Autodesk Fusion 360 part; units mm, degrees
(part 8 of 8)
  spline S32 degree 5 poles (83.4638, 120.4328) (83.5006, 120.4863) (83.5729, 120.594) (83.6772, 120.7581) (83.8082, 120.9817) (83.961, 121.2679) (84.106, 121.5588) (84.2462, 121.8526) (84.3838, 122.1479) (84.5197, 122.4443) (84.6536, 122.7417) (84.7851, 123.0405) (84.9132, 123.3412) (85.0374, 123.644) (85.1577, 123.949) (85.2744, 124.2559) (85.3881, 124.5645) (85.4991, 124.8744) (85.608, 125.1854) (85.7147, 125.4975) (85.8192, 125.8106) (85.9214, 126.1249) (86.0213, 126.4403) (86.1187, 126.757) (86.2136, 127.0748) (86.3062, 127.3938) (86.3966, 127.7138) (86.4849, 128.0348) (86.5711, 128.3567) (86.6553, 128.6794) (86.7376, 129.0031) (86.8178, 129.3277) (86.896, 129.6531) (86.9723, 129.9794) (87.0465, 130.3066) (87.1189, 130.6346) (87.1893, 130.9633) (87.2578, 131.2929) (87.3245, 131.6232) (87.3894, 131.9542) (87.4525, 132.286) (87.5137, 132.6184) (87.5732, 132.9516) (87.6309, 133.2854) (87.6869, 133.6199) (87.7411, 133.9551) (87.7935, 134.2909) (87.8443, 134.6274) (87.8933, 134.9645) (87.9407, 135.3021) (87.9864, 135.6404) (88.0305, 135.9792) (88.0729, 136.3187) (88.1136, 136.6587) (88.1527, 136.9992) (88.1902, 137.3403) (88.2261, 137.6819) (88.2604, 138.024) (88.2931, 138.3667) (88.3243, 138.7098) (88.3538, 139.0535) (88.3818, 139.3976) (88.4082, 139.7422) (88.4331, 140.0873) (88.4565, 140.4328) (88.4783, 140.7788) (88.4986, 141.1253) (88.5174, 141.4721) (88.5347, 141.8194) (88.5504, 142.1671) (88.5647, 142.5153) (88.575, 142.7941) (88.582, 143.0034) (88.5864, 143.143) (88.5885, 143.2129) knots 0 0 0 0 0 0 0.01428571 0.02857143 0.04285714 0.05714286 0.07142857 0.08571429 0.1 0.11428571 0.12857143 0.14285714 0.15714286 0.17142857 0.18571429 0.2 0.21428571 0.22857143 0.24285714 0.25714286 0.27142857 0.28571429 0.3 0.31428571 0.32857143 0.34285714 0.35714286 0.37142857 0.38571429 0.4 0.41428571 0.42857143 0.44285714 0.45714286 0.47142857 0.48571429 0.5 0.51428571 0.52857143 0.54285714 0.55714286 0.57142857 0.58571429 0.6 0.61428571 0.62857143 0.64285714 0.65714286 0.67142857 0.68571429 0.7 0.71428571 0.72857143 0.74285714 0.75714286 0.77142857 0.78571429 0.8 0.81428571 0.82857143 0.84285714 0.85714286 0.87142857 0.88571429 0.9 0.91428571 0.92857143 0.94285714 0.95714286 0.97142857 0.98571429 1 1 1 1 1 1
  arc A66 (88.5885, 143.2129) -> (80.7195, 147.756) centre (2.1352, 2.5578) ccw
  spline S33 degree 5 poles (80.7195, 147.756) (80.66, 147.7193) (80.5413, 147.6457) (80.3635, 147.535) (80.1272, 147.3867) (79.8328, 147.2003) (79.5396, 147.0127) (79.2475, 146.8241) (78.9565, 146.6344) (78.6666, 146.4436) (78.3779, 146.2517) (78.0903, 146.0587) (77.8039, 145.8646) (77.5187, 145.6694) (77.2347, 145.4731) (76.9518, 145.2757) (76.6702, 145.0772) (76.3898, 144.8775) (76.1107, 144.6768) (75.8328, 144.4749) (75.5561, 144.2718) (75.2808, 144.0677) (75.0067, 143.8624) (74.734, 143.656) (74.4625, 143.4484) (74.1924, 143.2397) (73.9237, 143.0298) (73.6563, 142.8188) (73.3903, 142.6066) (73.1257, 142.3933) (72.8626, 142.1788) (72.6008, 141.963) (72.3406, 141.7462) (72.0818, 141.5281) (71.8245, 141.3088) (71.5687, 141.0883) (71.3145, 140.8666) (71.0618, 140.6437) (70.8107, 140.4195) (70.5611, 140.1942) (70.3133, 139.9676) (70.0671, 139.7397) (69.8226, 139.5105) (69.5799, 139.28) (69.3389, 139.0483) (69.0997, 138.8152) (68.8623, 138.5809) (68.6266, 138.3452) (68.3928, 138.1083) (68.1608, 137.87) (67.9309, 137.6303) (67.7032, 137.3892) (67.4776, 137.1465) (67.2544, 136.9023) (67.0333, 136.6567) (66.8144, 136.4096) (66.5975, 136.1611) (66.3825, 135.9114) (66.1697, 135.6602) (65.9593, 135.4075) (65.7519, 135.153) (65.5479, 134.8963) (65.3477, 134.6373) (65.1514, 134.376) (64.9583, 134.1128) (64.7677, 133.8481) (64.579, 133.5822) (64.392, 133.3154) (64.2077, 133.0471) (64.0283, 132.776) (63.8569, 132.5006) (63.7287, 132.2754) (63.6387, 132.103) (63.5816, 131.9866) (63.5537, 131.9279) knots -1 -1 -1 -1 -1 -1 -0.98571429 -0.97142857 -0.95714286 -0.94285714 -0.92857143 -0.91428571 -0.9 -0.88571429 -0.87142857 -0.85714286 -0.84285714 -0.82857143 -0.81428571 -0.8 -0.78571429 -0.77142857 -0.75714286 -0.74285714 -0.72857143 -0.71428571 -0.7 -0.68571429 -0.67142857 -0.65714286 -0.64285714 -0.62857143 -0.61428571 -0.6 -0.58571429 -0.57142857 -0.55714286 -0.54285714 -0.52857143 -0.51428571 -0.5 -0.48571429 -0.47142857 -0.45714286 -0.44285714 -0.42857143 -0.41428571 -0.4 -0.38571429 -0.37142857 -0.35714286 -0.34285714 -0.32857143 -0.31428571 -0.3 -0.28571429 -0.27142857 -0.25714286 -0.24285714 -0.22857143 -0.21428571 -0.2 -0.18571429 -0.17142857 -0.15714286 -0.14285714 -0.12857143 -0.11428571 -0.1 -0.08571429 -0.07142857 -0.05714286 -0.04285714 -0.02857143 -0.01428571 0 0 0 0 0 0
  line L33 (63.5537, 131.9279) -> (61.6139, 127.8434)
  arc A67 (59.5156, 127.0826) -> (61.6139, 127.8434) centre (60.1799, 128.5244) ccw
  arc A68 (59.5156, 127.0826) -> (49.6135, 131.1842) centre (2.1352, 2.5578) ccw
  arc A69 (48.6677, 133.2059) -> (49.6135, 131.1842) centre (50.1633, 132.6735) ccw
  line L34 (48.6677, 133.2059) -> (50.1843, 137.4657)
  spline S34 degree 5 poles (50.1843, 137.4657) (50.2061, 137.5269) (50.248, 137.6496) (50.3062, 137.8351) (50.3749, 138.085) (50.4484, 138.401) (50.5132, 138.7195) (50.5726, 139.0396) (50.6291, 139.3605) (50.6836, 139.6819) (50.736, 140.0039) (50.7856, 140.3265) (50.8315, 140.6501) (50.8731, 140.9748) (50.9104, 141.3005) (50.9437, 141.6272) (50.9736, 141.9546) (51.0007, 142.2827) (51.0253, 142.6113) (51.0476, 142.9404) (51.0675, 143.2699) (51.085, 143.5999) (51.0998, 143.9305) (51.1119, 144.2615) (51.1213, 144.5931) (51.1282, 144.9252) (51.1327, 145.2576) (51.1349, 145.5905) (51.1349, 145.9238) (51.1327, 146.2574) (51.1284, 146.5913) (51.1219, 146.9256) (51.1132, 147.2602) (51.1024, 147.5951) (51.0894, 147.9303) (51.0744, 148.2658) (51.0573, 148.6016) (51.0383, 148.9377) (51.0172, 149.274) (50.9942, 149.6105) (50.9692, 149.9473) (50.9424, 150.2843) (50.9136, 150.6215) (50.8829, 150.9589) (50.8504, 151.2965) (50.816, 151.6343) (50.7797, 151.9722) (50.7417, 152.3104) (50.7018, 152.6486) (50.6602, 152.9871) (50.6168, 153.3256) (50.5716, 153.6643) (50.5247, 154.0032) (50.4761, 154.3421) (50.4258, 154.6812) (50.3737, 155.0203) (50.32, 155.3596) (50.2645, 155.699) (50.2074, 156.0384) (50.1487, 156.3779) (50.0883, 156.7175) (50.0263, 157.0572) (49.9626, 157.3969) (49.8973, 157.7366) (49.8305, 158.0765) (49.762, 158.4163) (49.6919, 158.7562) (49.6203, 159.0961) (49.5471, 159.436) (49.4724, 159.776) (49.3961, 160.1159) (49.3338, 160.3879) (49.2864, 160.5919) (49.2545, 160.7279) (49.2384, 160.7959) knots 0 0 0 0 0 0 0.01428571 0.02857143 0.04285714 0.05714286 0.07142857 0.08571429 0.1 0.11428571 0.12857143 0.14285714 0.15714286 0.17142857 0.18571429 0.2 0.21428571 0.22857143 0.24285714 0.25714286 0.27142857 0.28571429 0.3 0.31428571 0.32857143 0.34285714 0.35714286 0.37142857 0.38571429 0.4 0.41428571 0.42857143 0.44285714 0.45714286 0.47142857 0.48571429 0.5 0.51428571 0.52857143 0.54285714 0.55714286 0.57142857 0.58571429 0.6 0.61428571 0.62857143 0.64285714 0.65714286 0.67142857 0.68571429 0.7 0.71428571 0.72857143 0.74285714 0.75714286 0.77142857 0.78571429 0.8 0.81428571 0.82857143 0.84285714 0.85714286 0.87142857 0.88571429 0.9 0.91428571 0.92857143 0.94285714 0.95714286 0.97142857 0.98571429 1 1 1 1 1 1
  arc A70 (49.2384, 160.7959) -> (40.4617, 163.1476) centre (2.1352, 2.5578) ccw
  spline S35 degree 5 poles (40.4617, 163.1476) (40.4138, 163.0968) (40.3182, 162.9949) (40.1751, 162.842) (39.9852, 162.6376) (39.7491, 162.3813) (39.5144, 162.1243) (39.2811, 161.8665) (39.0491, 161.6079) (38.8185, 161.3486) (38.5893, 161.0885) (38.3614, 160.8277) (38.135, 160.5661) (37.91, 160.3037) (37.6865, 160.0406) (37.4644, 159.7767) (37.2438, 159.512) (37.0246, 159.2466) (36.8069, 158.9804) (36.5907, 158.7135) (36.3761, 158.4458) (36.1629, 158.1773) (35.9514, 157.9081) (35.7413, 157.6381) (35.5329, 157.3674) (35.326, 157.0959) (35.1207, 156.8236) (34.9171, 156.5506) (34.7151, 156.2768) (34.5147, 156.0022) (34.316, 155.7269) (34.119, 155.4508) (33.9238, 155.1739) (33.7302, 154.8963) (33.5385, 154.6179) (33.3485, 154.3387) (33.1603, 154.0587) (32.9739, 153.778) (32.7893, 153.4965) (32.6067, 153.2143) (32.4259, 152.9312) (32.2471, 152.6474) (32.0702, 152.3627) (31.8954, 152.0773) (31.7227, 151.791) (31.5519, 151.504) (31.3832, 151.2162) (31.2166, 150.9276) (31.0521, 150.6382) (30.8897, 150.3481) (30.7297, 150.057) (30.5721, 149.7652) (30.417, 149.4724) (30.2646, 149.1787) (30.1146, 148.8842) (29.9671, 148.5889) (29.8219, 148.2928) (29.6789, 147.9959) (29.5383, 147.6982) (29.4005, 147.3997) (29.266, 147.1001) (29.1355, 146.7994) (29.0091, 146.4974) (28.8871, 146.1942) (28.7687, 145.89) (28.6532, 145.5849) (28.5397, 145.2793) (28.4281, 144.9732) (28.3195, 144.6663) (28.2164, 144.3581) (28.1221, 144.0477) (28.0566, 143.7969) (28.0142, 143.6072) (27.9892, 143.4799) (27.9775, 143.416) knots -1 -1 -1 -1 -1 -1 -0.98571429 -0.97142857 -0.95714286 -0.94285714 -0.92857143 -0.91428571 -0.9 -0.88571429 -0.87142857 -0.85714286 -0.84285714 -0.82857143 -0.81428571 -0.8 -0.78571429 -0.77142857 -0.75714286 -0.74285714 -0.72857143 -0.71428571 -0.7 -0.68571429 -0.67142857 -0.65714286 -0.64285714 -0.62857143 -0.61428571 -0.6 -0.58571429 -0.57142857 -0.55714286 -0.54285714 -0.52857143 -0.51428571 -0.5 -0.48571429 -0.47142857 -0.45714286 -0.44285714 -0.42857143 -0.41428571 -0.4 -0.38571429 -0.37142857 -0.35714286 -0.34285714 -0.32857143 -0.31428571 -0.3 -0.28571429 -0.27142857 -0.25714286 -0.24285714 -0.22857143 -0.21428571 -0.2 -0.18571429 -0.17142857 -0.15714286 -0.14285714 -0.12857143 -0.11428571 -0.1 -0.08571429 -0.07142857 -0.05714286 -0.04285714 -0.02857143 -0.01428571 0 0 0 0 0 0
  line L35 (27.9775, 143.416) -> (27.1609, 138.9686)
  arc A71 (25.331, 137.6907) -> (27.1609, 138.9686) centre (25.5995, 139.2553) ccw
  arc A72 (25.331, 137.6907) -> (14.7048, 139.0896) centre (2.1352, 2.5578) ccw
  arc A73 (13.2679, 140.7977) -> (14.7048, 139.0896) centre (14.8503, 140.6704) ccw
  line L36 (13.2679, 140.7977) -> (13.6303, 145.3049)
  spline S36 degree 5 poles (13.6303, 145.3049) (13.6355, 145.3696) (13.6443, 145.499) (13.6525, 145.6932) (13.6541, 145.9524) (13.6434, 146.2766) (13.6235, 146.6011) (13.598, 146.9256) (13.5696, 147.2502) (13.539, 147.5748) (13.5063, 147.8993) (13.4707, 148.2238) (13.4313, 148.5483) (13.3875, 148.8726) (13.3392, 149.1969) (13.2868, 149.5211) (13.231, 149.8451) (13.1722, 150.169) (13.1109, 150.4928) (13.0473, 150.8164) (12.9813, 151.1399) (12.9127, 151.4631) (12.8414, 151.7863) (12.7674, 152.1092) (12.6907, 152.4319) (12.6115, 152.7544) (12.5297, 153.0768) (12.4457, 153.3989) (12.3594, 153.7207) (12.271, 154.0424) (12.1804, 154.3638) (12.0876, 154.685) (11.9926, 155.006) (11.8955, 155.3267) (11.7962, 155.6472) (11.6948, 155.9673) (11.5914, 156.2873) (11.486, 156.6069) (11.3786, 156.9263) (11.2693, 157.2455) (11.158, 157.5643) (11.0449, 157.8829) (10.9298, 158.2011) (10.8129, 158.5191) (10.694, 158.8368) (10.5734, 159.1541) (10.4509, 159.4712) (10.3267, 159.7879) (10.2006, 160.1044) (10.0728, 160.4205) (9.9433, 160.7363) (9.812, 161.0518) (9.679, 161.3669) (9.5443, 161.6817) (9.4079, 161.9962) (9.2698, 162.3104) (9.1301, 162.6241) (8.9887, 162.9376) (8.8457, 163.2507) (8.7011, 163.5634) (8.5549, 163.8758) (8.407, 164.1878) (8.2576, 164.4995) (8.1066, 164.8108) (7.9541, 165.1217) (7.8, 165.4323) (7.6444, 165.7424) (7.4872, 166.0522) (7.3285, 166.3616) (7.1683, 166.6706) (7.0066, 166.9793) (6.8761, 167.2259) (6.7775, 167.4106) (6.7115, 167.5338) (6.6784, 167.5953) knots 0 0 0 0 0 0 0.01428571 0.02857143 0.04285714 0.05714286 0.07142857 0.08571429 0.1 0.11428571 0.12857143 0.14285714 0.15714286 0.17142857 0.18571429 0.2 0.21428571 0.22857143 0.24285714 0.25714286 0.27142857 0.28571429 0.3 0.31428571 0.32857143 0.34285714 0.35714286 0.37142857 0.38571429 0.4 0.41428571 0.42857143 0.44285714 0.45714286 0.47142857 0.48571429 0.5 0.51428571 0.52857143 0.54285714 0.55714286 0.57142857 0.58571429 0.6 0.61428571 0.62857143 0.64285714 0.65714286 0.67142857 0.68571429 0.7 0.71428571 0.72857143 0.74285714 0.75714286 0.77142857 0.78571429 0.8 0.81428571 0.82857143 0.84285714 0.85714286 0.87142857 0.88571429 0.9 0.91428571 0.92857143 0.94285714 0.95714286 0.97142857 0.98571429 1 1 1 1 1 1
  arc A74 (6.6784, 167.5953) -> (-2.4079, 167.5953) centre (2.1352, 2.5578) ccw
  spline S37 degree 5 poles (-2.4079, 167.5953) (-2.441, 167.5338) (-2.5071, 167.4106) (-2.6056, 167.2259) (-2.7362, 166.9793) (-2.8979, 166.6706) (-3.0581, 166.3616) (-3.2167, 166.0522) (-3.3739, 165.7424) (-3.5295, 165.4323) (-3.6836, 165.1217) (-3.8362, 164.8108) (-3.9872, 164.4995) (-4.1366, 164.1878) (-4.2844, 163.8758) (-4.4306, 163.5634) (-4.5753, 163.2507) (-4.7183, 162.9376) (-4.8596, 162.6241) (-4.9994, 162.3104) (-5.1374, 161.9962) (-5.2738, 161.6817) (-5.4085, 161.3669) (-5.5415, 161.0518) (-5.6728, 160.7363) (-5.8024, 160.4205) (-5.9302, 160.1044) (-6.0562, 159.7879) (-6.1805, 159.4712) (-6.3029, 159.1541) (-6.4236, 158.8368) (-6.5424, 158.5191) (-6.6594, 158.2011) (-6.7744, 157.8829) (-6.8876, 157.5643) (-6.9989, 157.2455) (-7.1082, 156.9263) (-7.2156, 156.6069) (-7.321, 156.2873) (-7.4244, 155.9673) (-7.5257, 155.6472) (-7.625, 155.3267) (-7.7221, 155.006) (-7.8171, 154.685) (-7.9099, 154.3638) (-8.0005, 154.0424) (-8.089, 153.7207) (-8.1753, 153.3989) (-8.2593, 153.0768) (-8.341, 152.7544) (-8.4203, 152.4319) (-8.497, 152.1092) (-8.571, 151.7863) (-8.6422, 151.4631) (-8.7108, 151.1399) (-8.7768, 150.8164) (-8.8405, 150.4928) (-8.9017, 150.169) (-8.9605, 149.8451) (-9.0164, 149.5211) (-9.0687, 149.1969) (-9.117, 148.8726) (-9.1609, 148.5483) (-9.2003, 148.2238) (-9.2359, 147.8993) (-9.2686, 147.5748) (-9.2991, 147.2502) (-9.3276, 146.9256) (-9.3531, 146.6011) (-9.3729, 146.2766) (-9.3837, 145.9524) (-9.382, 145.6932) (-9.3738, 145.499) (-9.3651, 145.3696) (-9.3599, 145.3049) knots -1 -1 -1 -1 -1 -1 -0.98571429 -0.97142857 -0.95714286 -0.94285714 -0.92857143 -0.91428571 -0.9 -0.88571429 -0.87142857 -0.85714286 -0.84285714 -0.82857143 -0.81428571 -0.8 -0.78571429 -0.77142857 -0.75714286 -0.74285714 -0.72857143 -0.71428571 -0.7 -0.68571429 -0.67142857 -0.65714286 -0.64285714 -0.62857143 -0.61428571 -0.6 -0.58571429 -0.57142857 -0.55714286 -0.54285714 -0.52857143 -0.51428571 -0.5 -0.48571429 -0.47142857 -0.45714286 -0.44285714 -0.42857143 -0.41428571 -0.4 -0.38571429 -0.37142857 -0.35714286 -0.34285714 -0.32857143 -0.31428571 -0.3 -0.28571429 -0.27142857 -0.25714286 -0.24285714 -0.22857143 -0.21428571 -0.2 -0.18571429 -0.17142857 -0.15714286 -0.14285714 -0.12857143 -0.11428571 -0.1 -0.08571429 -0.07142857 -0.05714286 -0.04285714 -0.02857143 -0.01428571 0 0 0 0 0 0
  line L37 (-9.3599, 145.3049) -> (-8.9975, 140.7977)
  arc A75 (-10.4344, 139.0896) -> (-8.9975, 140.7977) centre (-10.5799, 140.6704) ccw
  arc A76 (-10.4344, 139.0896) -> (-21.0605, 137.6907) centre (2.1352, 2.5578) ccw
  arc A77 (-22.8905, 138.9686) -> (-21.0605, 137.6907) centre (-21.3291, 139.2553) ccw
  line L38 (-22.8905, 138.9686) -> (-23.707, 143.416)
  spline S38 degree 5 poles (-23.707, 143.416) (-23.7188, 143.4799) (-23.7438, 143.6072) (-23.7861, 143.7969) (-23.8516, 144.0477) (-23.9459, 144.3581) (-24.0491, 144.6663) (-24.1577, 144.9732) (-24.2692, 145.2793) (-24.3827, 145.5849) (-24.4983, 145.89) (-24.6166, 146.1942) (-24.7387, 146.4974) (-24.865, 146.7994) (-24.9956, 147.1001) (-25.1301, 147.3997) (-25.2679, 147.6982) (-25.4085, 147.9959) (-25.5515, 148.2928) (-25.6967, 148.5889) (-25.8442, 148.8842) (-25.9941, 149.1787) (-26.1466, 149.4724) (-26.3016, 149.7652) (-26.4592, 150.057) (-26.6192, 150.3481) (-26.7816, 150.6382) (-26.9462, 150.9276) (-27.1128, 151.2162) (-27.2815, 151.504) (-27.4522, 151.791) (-27.625, 152.0773) (-27.7998, 152.3627) (-27.9766, 152.6474) (-28.1554, 152.9312) (-28.3362, 153.2143) (-28.5189, 153.4965) (-28.7035, 153.778) (-28.8898, 154.0587) (-29.078, 154.3387) (-29.268, 154.6179) (-29.4598, 154.8963) (-29.6533, 155.1739) (-29.8486, 155.4508) (-30.0456, 155.7269) (-30.2442, 156.0022) (-30.4446, 156.2768) (-30.6466, 156.5506) (-30.8503, 156.8236) (-31.0555, 157.0959) (-31.2624, 157.3674) (-31.4709, 157.6381) (-31.6809, 157.9081) (-31.8925, 158.1773) (-32.1056, 158.4458) (-32.3203, 158.7135) (-32.5365, 158.9804) (-32.7541, 159.2466) (-32.9733, 159.512) (-33.1939, 159.7767) (-33.416, 160.0406) (-33.6396, 160.3037) (-33.8646, 160.5661) (-34.091, 160.8277) (-34.3188, 161.0885) (-34.548, 161.3486) (-34.7786, 161.6079) (-35.0106, 161.8665) (-35.244, 162.1243) (-35.4787, 162.3813) (-35.7148, 162.6376) (-35.9047, 162.842) (-36.0477, 162.9949) (-36.1434, 163.0968) (-36.1913, 163.1476) knots 0 0 0 0 0 0 0.01428571 0.02857143 0.04285714 0.05714286 0.07142857 0.08571429 0.1 0.11428571 0.12857143 0.14285714 0.15714286 0.17142857 0.18571429 0.2 0.21428571 0.22857143 0.24285714 0.25714286 0.27142857 0.28571429 0.3 0.31428571 0.32857143 0.34285714 0.35714286 0.37142857 0.38571429 0.4 0.41428571 0.42857143 0.44285714 0.45714286 0.47142857 0.48571429 0.5 0.51428571 0.52857143 0.54285714 0.55714286 0.57142857 0.58571429 0.6 0.61428571 0.62857143 0.64285714 0.65714286 0.67142857 0.68571429 0.7 0.71428571 0.72857143 0.74285714 0.75714286 0.77142857 0.78571429 0.8 0.81428571 0.82857143 0.84285714 0.85714286 0.87142857 0.88571429 0.9 0.91428571 0.92857143 0.94285714 0.95714286 0.97142857 0.98571429 1 1 1 1 1 1
  arc A78 (-36.1913, 163.1476) -> (-44.968, 160.7959) centre (2.1352, 2.5578) ccw
  spline S39 degree 5 poles (-44.968, 160.7959) (-44.984, 160.7279) (-45.0159, 160.5919) (-45.0633, 160.3879) (-45.1256, 160.1159) (-45.2019, 159.776) (-45.2767, 159.436) (-45.3499, 159.0961) (-45.4215, 158.7562) (-45.4915, 158.4163) (-45.56, 158.0765) (-45.6269, 157.7366) (-45.6922, 157.3969) (-45.7558, 157.0572) (-45.8178, 156.7175) (-45.8782, 156.3779) (-45.937, 156.0384) (-45.9941, 155.699) (-46.0495, 155.3596) (-46.1033, 155.0203) (-46.1553, 154.6812) (-46.2057, 154.3421) (-46.2543, 154.0032) (-46.3012, 153.6643) (-46.3464, 153.3256) (-46.3898, 152.9871) (-46.4314, 152.6486) (-46.4712, 152.3104) (-46.5093, 151.9722) (-46.5455, 151.6343) (-46.5799, 151.2965) (-46.6125, 150.9589) (-46.6431, 150.6215) (-46.6719, 150.2843) (-46.6988, 149.9473) (-46.7237, 149.6105) (-46.7467, 149.274) (-46.7678, 148.9377) (-46.7869, 148.6016) (-46.804, 148.2658) (-46.819, 147.9303) (-46.8319, 147.5951) (-46.8427, 147.2602) (-46.8514, 146.9256) (-46.8579, 146.5913) (-46.8623, 146.2574) (-46.8644, 145.9238) (-46.8645, 145.5905) (-46.8623, 145.2576) (-46.8578, 144.9252) (-46.8509, 144.5931) (-46.8414, 144.2615) (-46.8293, 143.9305) (-46.8145, 143.5999) (-46.7971, 143.2699) (-46.7772, 142.9404) (-46.7549, 142.6113) (-46.7303, 142.2827) (-46.7032, 141.9546) (-46.6733, 141.6272) (-46.6399, 141.3005) (-46.6027, 140.9748) (-46.5611, 140.6501) (-46.5152, 140.3265) (-46.4656, 140.0039) (-46.4131, 139.6819) (-46.3586, 139.3605) (-46.3021, 139.0396) (-46.2427, 138.7195) (-46.178, 138.401) (-46.1044, 138.085) (-46.0358, 137.8351) (-45.9776, 137.6496) (-45.9356, 137.5269) (-45.9138, 137.4657) knots -1 -1 -1 -1 -1 -1 -0.98571429 -0.97142857 -0.95714286 -0.94285714 -0.92857143 -0.91428571 -0.9 -0.88571429 -0.87142857 -0.85714286 -0.84285714 -0.82857143 -0.81428571 -0.8 -0.78571429 -0.77142857 -0.75714286 -0.74285714 -0.72857143 -0.71428571 -0.7 -0.68571429 -0.67142857 -0.65714286 -0.64285714 -0.62857143 -0.61428571 -0.6 -0.58571429 -0.57142857 -0.55714286 -0.54285714 -0.52857143 -0.51428571 -0.5 -0.48571429 -0.47142857 -0.45714286 -0.44285714 -0.42857143 -0.41428571 -0.4 -0.38571429 -0.37142857 -0.35714286 -0.34285714 -0.32857143 -0.31428571 -0.3 -0.28571429 -0.27142857 -0.25714286 -0.24285714 -0.22857143 -0.21428571 -0.2 -0.18571429 -0.17142857 -0.15714286 -0.14285714 -0.12857143 -0.11428571 -0.1 -0.08571429 -0.07142857 -0.05714286 -0.04285714 -0.02857143 -0.01428571 0 0 0 0 0 0
  line L39 (-45.9138, 137.4657) -> (-44.3973, 133.2059)
  arc A79 (-45.3431, 131.1842) -> (-44.3973, 133.2059) centre (-45.8928, 132.6735) ccw
  arc A80 (-45.3431, 131.1842) -> (-55.2451, 127.0826) centre (2.1352, 2.5578) ccw
  arc A81 (-57.3435, 127.8434) -> (-55.2451, 127.0826) centre (-55.9095, 128.5244) ccw
  line L40 (-57.3435, 127.8434) -> (-59.2833, 131.9279)
  spline S40 degree 5 poles (-59.2833, 131.9279) (-59.3111, 131.9866) (-59.3682, 132.103) (-59.4582, 132.2754) (-59.5864, 132.5006) (-59.7578, 132.776) (-59.9373, 133.0471) (-60.1216, 133.3154) (-60.3085, 133.5822) (-60.4973, 133.8481) (-60.6879, 134.1128) (-60.8809, 134.376) (-61.0773, 134.6373) (-61.2775, 134.8963) (-61.4814, 135.153) (-61.6889, 135.4075) (-61.8992, 135.6602) (-62.1121, 135.9114) (-62.327, 136.1611) (-62.544, 136.4096) (-62.7629, 136.6567) (-62.9839, 136.9023) (-63.2072, 137.1465) (-63.4327, 137.3892) (-63.6605, 137.6303) (-63.8904, 137.87) (-64.1223, 138.1083) (-64.3562, 138.3452) (-64.5918, 138.5809) (-64.8293, 138.8152) (-65.0685, 139.0483) (-65.3094, 139.28) (-65.5521, 139.5105) (-65.7966, 139.7397) (-66.0428, 139.9676) (-66.2907, 140.1942) (-66.5402, 140.4195) (-66.7913, 140.6437) (-67.044, 140.8666) (-67.2983, 141.0883) (-67.554, 141.3088) (-67.8113, 141.5281) (-68.0701, 141.7462) (-68.3304, 141.963) (-68.5921, 142.1788) (-68.8553, 142.3933) (-69.1199, 142.6066) (-69.3859, 142.8188) (-69.6532, 143.0298) (-69.922, 143.2397) (-70.1921, 143.4484) (-70.4635, 143.656) (-70.7363, 143.8624) (-71.0103, 144.0677) (-71.2857, 144.2718) (-71.5623, 144.4749) (-71.8402, 144.6768) (-72.1194, 144.8775) (-72.3998, 145.0772) (-72.6814, 145.2757) (-72.9642, 145.4731) (-73.2482, 145.6694) (-73.5335, 145.8646) (-73.8199, 146.0587) (-74.1074, 146.2517) (-74.3962, 146.4436) (-74.686, 146.6344) (-74.977, 146.8241) (-75.2692, 147.0127) (-75.5624, 147.2003) (-75.8567, 147.3867) (-76.0931, 147.535) (-76.2709, 147.6457) (-76.3896, 147.7193) (-76.449, 147.756) knots 0 0 0 0 0 0 0.01428571 0.02857143 0.04285714 0.05714286 0.07142857 0.08571429 0.1 0.11428571 0.12857143 0.14285714 0.15714286 0.17142857 0.18571429 0.2 0.21428571 0.22857143 0.24285714 0.25714286 0.27142857 0.28571429 0.3 0.31428571 0.32857143 0.34285714 0.35714286 0.37142857 0.38571429 0.4 0.41428571 0.42857143 0.44285714 0.45714286 0.47142857 0.48571429 0.5 0.51428571 0.52857143 0.54285714 0.55714286 0.57142857 0.58571429 0.6 0.61428571 0.62857143 0.64285714 0.65714286 0.67142857 0.68571429 0.7 0.71428571 0.72857143 0.74285714 0.75714286 0.77142857 0.78571429 0.8 0.81428571 0.82857143 0.84285714 0.85714286 0.87142857 0.88571429 0.9 0.91428571 0.92857143 0.94285714 0.95714286 0.97142857 0.98571429 1 1 1 1 1 1
  arc A82 (-76.449, 147.756) -> (-84.318, 143.2129) centre (2.1352, 2.5578) ccw
  spline S41 degree 5 poles (-84.318, 143.2129) (-84.3159, 143.143) (-84.3115, 143.0034) (-84.3045, 142.7941) (-84.2943, 142.5153) (-84.28, 142.1671) (-84.2642, 141.8194) (-84.2469, 141.4721) (-84.2281, 141.1253) (-84.2078, 140.7788) (-84.186, 140.4328) (-84.1627, 140.0873) (-84.1378, 139.7422) (-84.1113, 139.3976) (-84.0834, 139.0535) (-84.0538, 138.7098) (-84.0227, 138.3667) (-83.99, 138.024) (-83.9557, 137.6819) (-83.9198, 137.3403) (-83.8823, 136.9992) (-83.8432, 136.6587) (-83.8024, 136.3187) (-83.76, 135.9792) (-83.716, 135.6404) (-83.6703, 135.3021) (-83.6229, 134.9645) (-83.5738, 134.6274) (-83.5231, 134.2909) (-83.4706, 133.9551) (-83.4164, 133.6199) (-83.3605, 133.2854) (-83.3028, 132.9516) (-83.2433, 132.6184) (-83.182, 132.286) (-83.1189, 131.9542) (-83.0541, 131.6232) (-82.9874, 131.2929) (-82.9188, 130.9633) (-82.8484, 130.6346) (-82.7761, 130.3066) (-82.7018, 129.9794) (-82.6256, 129.6531) (-82.5474, 129.3277) (-82.4671, 129.0031) (-82.3849, 128.6794) (-82.3007, 128.3567) (-82.2144, 128.0348) (-82.1262, 127.7138) (-82.0358, 127.3938) (-81.9432, 127.0748) (-81.8482, 126.757) (-81.7508, 126.4403) (-81.651, 126.1249) (-81.5487, 125.8106) (-81.4442, 125.4975) (-81.3375, 125.1854) (-81.2287, 124.8744) (-81.1176, 124.5645) (-81.004, 124.2559) (-80.8872, 123.949) (-80.7669, 123.644) (-80.6427, 123.3412) (-80.5146, 123.0405) (-80.3832, 122.7417) (-80.2492, 122.4443) (-80.1134, 122.1479) (-79.9758, 121.8526) (-79.8355, 121.5588) (-79.6905, 121.2679) (-79.5377, 120.9817) (-79.4067, 120.7581) (-79.3025, 120.594) (-79.2302, 120.4863) (-79.1933, 120.4328) knots -1 -1 -1 -1 -1 -1 -0.98571429 -0.97142857 -0.95714286 -0.94285714 -0.92857143 -0.91428571 -0.9 -0.88571429 -0.87142857 -0.85714286 -0.84285714 -0.82857143 -0.81428571 -0.8 -0.78571429 -0.77142857 -0.75714286 -0.74285714 -0.72857143 -0.71428571 -0.7 -0.68571429 -0.67142857 -0.65714286 -0.64285714 -0.62857143 -0.61428571 -0.6 -0.58571429 -0.57142857 -0.55714286 -0.54285714 -0.52857143 -0.51428571 -0.5 -0.48571429 -0.47142857 -0.45714286 -0.44285714 -0.42857143 -0.41428571 -0.4 -0.38571429 -0.37142857 -0.35714286 -0.34285714 -0.32857143 -0.31428571 -0.3 -0.28571429 -0.27142857 -0.25714286 -0.24285714 -0.22857143 -0.21428571 -0.2 -0.18571429 -0.17142857 -0.15714286 -0.14285714 -0.12857143 -0.11428571 -0.1 -0.08571429 -0.07142857 -0.05714286 -0.04285714 -0.02857143 -0.01428571 0 0 0 0 0 0
  line L41 (-79.1933, 120.4328) -> (-76.6259, 116.7107)
  arc A83 (-77.0163, 114.513) -> (-76.6259, 116.7107) centre (-77.9327, 115.8093) ccw
  arc A84 (-77.0163, 114.513) -> (-85.5193, 107.9884) centre (2.1352, 2.5578) ccw
  arc A85 (-87.7431, 108.1802) -> (-85.5193, 107.9884) centre (-86.5342, 109.2091) ccw
  line L42 (-87.7431, 108.1802) -> (-90.6739, 111.6235)
  spline S42 degree 5 poles (-90.6739, 111.6235) (-90.716, 111.6729) (-90.8013, 111.7706) (-90.9329, 111.9138) (-91.115, 112.0982) (-91.3518, 112.3199) (-91.5953, 112.5352) (-91.8428, 112.7467) (-92.0924, 112.956) (-92.3435, 113.164) (-92.5961, 113.3704) (-92.8508, 113.5746) (-93.1081, 113.7762) (-93.3684, 113.9745) (-93.6319, 114.1697) (-93.8981, 114.3619) (-94.1668, 114.5515) (-94.4374, 114.739) (-94.7096, 114.9246) (-94.9834, 115.1085) (-95.2589, 115.2905) (-95.5359, 115.4706) (-95.8148, 115.6487) (-96.0955, 115.8247) (-96.3779, 115.9987) (-96.662, 116.1707) (-96.9477, 116.3408) (-97.2349, 116.5091) (-97.5235, 116.6758) (-97.8135, 116.8407) (-98.1049, 117.0039) (-98.3976, 117.1654) (-98.6917, 117.3252) (-98.9872, 117.4832) (-99.284, 117.6397) (-99.582, 117.7944) (-99.8814, 117.9475) (-100.182, 118.099) (-100.4837, 118.2489) (-100.7867, 118.3973) (-101.0908, 118.544) (-101.3961, 118.6893) (-101.7025, 118.833) (-102.01, 118.9751) (-102.3187, 119.1157) (-102.6284, 119.2548) (-102.9392, 119.3924) (-103.2511, 119.5285) (-103.5639, 119.6631) (-103.8778, 119.7963) (-104.1928, 119.928) (-104.5087, 120.0582) (-104.8255, 120.187) (-105.1434, 120.3144) (-105.4622, 120.4403) (-105.782, 120.5648) (-106.1027, 120.6879) (-106.4243, 120.8096) (-106.7468, 120.9299) (-107.0702, 121.0487) (-107.3945, 121.1662) (-107.7196, 121.2823) (-108.0457, 121.3971) (-108.3725, 121.5104) (-108.7003, 121.6224) (-109.0288, 121.733) (-109.3582, 121.8423) (-109.6884, 121.9502) (-110.0194, 122.0568) (-110.3511, 122.1621) (-110.6837, 122.266) (-110.9504, 122.348) (-111.1507, 122.409) (-111.2845, 122.4493) (-111.3514, 122.4694) knots 0 0 0 0 0 0 0.01428571 0.02857143 0.04285714 0.05714286 0.07142857 0.08571429 0.1 0.11428571 0.12857143 0.14285714 0.15714286 0.17142857 0.18571429 0.2 0.21428571 0.22857143 0.24285714 0.25714286 0.27142857 0.28571429 0.3 0.31428571 0.32857143 0.34285714 0.35714286 0.37142857 0.38571429 0.4 0.41428571 0.42857143 0.44285714 0.45714286 0.47142857 0.48571429 0.5 0.51428571 0.52857143 0.54285714 0.55714286 0.57142857 0.58571429 0.6 0.61428571 0.62857143 0.64285714 0.65714286 0.67142857 0.68571429 0.7 0.71428571 0.72857143 0.74285714 0.75714286 0.77142857 0.78571429 0.8 0.81428571 0.82857143 0.84285714 0.85714286 0.87142857 0.88571429 0.9 0.91428571 0.92857143 0.94285714 0.95714286 0.97142857 0.98571429 1 1 1 1 1 1
  arc A86 (-111.3514, 122.4694) -> (-117.7764, 116.0444) centre (2.1352, 2.5578) ccw
  spline S43 degree 5 poles (-117.7764, 116.0444) (-117.7563, 115.9775) (-117.7159, 115.8438) (-117.655, 115.6434) (-117.5729, 115.3767) (-117.469, 115.0442) (-117.3638, 114.7124) (-117.2572, 114.3814) (-117.1493, 114.0512) (-117.04, 113.7218) (-116.9294, 113.3933) (-116.8174, 113.0656) (-116.704, 112.7387) (-116.5893, 112.4127) (-116.4732, 112.0875) (-116.3557, 111.7632) (-116.2368, 111.4398) (-116.1166, 111.1173) (-115.9949, 110.7957) (-115.8718, 110.475) (-115.7473, 110.1552) (-115.6214, 109.8364) (-115.494, 109.5186) (-115.3652, 109.2017) (-115.235, 108.8858) (-115.1033, 108.5709) (-114.9701, 108.257) (-114.8355, 107.9441) (-114.6994, 107.6322) (-114.5618, 107.3214) (-114.4227, 107.0117) (-114.2821, 106.7031) (-114.1399, 106.3955) (-113.9962, 106.0891) (-113.851, 105.7839) (-113.7042, 105.4797) (-113.5559, 105.1768) (-113.406, 104.875) (-113.2545, 104.5744) (-113.1014, 104.2751) (-112.9466, 103.977) (-112.7902, 103.6802) (-112.6321, 103.3847) (-112.4723, 103.0906) (-112.3108, 102.7979) (-112.1476, 102.5065) (-111.9827, 102.2165) (-111.8161, 101.9279) (-111.6478, 101.6407) (-111.4777, 101.355) (-111.3056, 101.0709) (-111.1317, 100.7885) (-110.9556, 100.5078) (-110.7776, 100.229) (-110.5975, 99.9519) (-110.4154, 99.6765) (-110.2316, 99.4026) (-110.046, 99.1304) (-109.8585, 98.8598) (-109.6688, 98.5912) (-109.4767, 98.3249) (-109.2815, 98.0615) (-109.0832, 97.8011) (-108.8816, 97.5438) (-108.6773, 97.2892) (-108.4709, 97.0366) (-108.263, 96.7855) (-108.0536, 96.5358) (-107.8422, 96.2883) (-107.6268, 96.0449) (-107.4052, 95.808) (-107.2207, 95.6259) (-107.0776, 95.4944) (-106.9799, 95.409) (-106.9304, 95.367) knots -1 -1 -1 -1 -1 -1 -0.98571429 -0.97142857 -0.95714286 -0.94285714 -0.92857143 -0.91428571 -0.9 -0.88571429 -0.87142857 -0.85714286 -0.84285714 -0.82857143 -0.81428571 -0.8 -0.78571429 -0.77142857 -0.75714286 -0.74285714 -0.72857143 -0.71428571 -0.7 -0.68571429 -0.67142857 -0.65714286 -0.64285714 -0.62857143 -0.61428571 -0.6 -0.58571429 -0.57142857 -0.55714286 -0.54285714 -0.52857143 -0.51428571 -0.5 -0.48571429 -0.47142857 -0.45714286 -0.44285714 -0.42857143 -0.41428571 -0.4 -0.38571429 -0.37142857 -0.35714286 -0.34285714 -0.32857143 -0.31428571 -0.3 -0.28571429 -0.27142857 -0.25714286 -0.24285714 -0.22857143 -0.21428571 -0.2 -0.18571429 -0.17142857 -0.15714286 -0.14285714 -0.12857143 -0.11428571 -0.1 -0.08571429 -0.07142857 -0.05714286 -0.04285714 -0.02857143 -0.01428571 0 0 0 0 0 0
  line L43 (-106.9304, 95.367) -> (-103.4871, 92.4361)
  arc A87 (-103.2954, 90.2123) -> (-103.4871, 92.4361) centre (-104.5161, 91.2272) ccw
  arc A88 (-103.2954, 90.2123) -> (-109.82, 81.7093) centre (2.1352, 2.5578) ccw
  arc A89 (-112.0176, 81.319) -> (-109.82, 81.7093) centre (-111.1163, 82.6257) ccw
  line L44 (-112.0176, 81.319) -> (-115.7398, 83.8864)
  spline S44 degree 5 poles (-115.7398, 83.8864) (-115.7932, 83.9232) (-115.901, 83.9955) (-116.0651, 84.0998) (-116.2887, 84.2308) (-116.5749, 84.3836) (-116.8657, 84.5286) (-117.1595, 84.6688) (-117.4549, 84.8064) (-117.7512, 84.9423) (-118.0487, 85.0762) (-118.3475, 85.2077) (-118.6482, 85.3357) (-118.951, 85.4599) (-119.256, 85.5802) (-119.5629, 85.697) (-119.8715, 85.8106) (-120.1814, 85.9217) (-120.4924, 86.0305) (-120.8045, 86.1372) (-121.1176, 86.2418) (-121.4319, 86.344) (-121.7473, 86.4439) (-122.064, 86.5412) (-122.3818, 86.6362) (-122.7007, 86.7288) (-123.0207, 86.8192) (-123.3417, 86.9075) (-123.6636, 86.9937) (-123.9864, 87.0779) (-124.3101, 87.1602) (-124.6347, 87.2404) (-124.9601, 87.3186) (-125.2864, 87.3949) (-125.6136, 87.4691) (-125.9415, 87.5414) (-126.2703, 87.6119) (-126.5999, 87.6804) (-126.9301, 87.7471) (-127.2612, 87.812) (-127.5929, 87.875) (-127.9254, 87.9363) (-128.2585, 87.9958) (-128.5924, 88.0535) (-128.9269, 88.1094) (-129.2621, 88.1636) (-129.5979, 88.2161) (-129.9344, 88.2669) (-130.2714, 88.3159) (-130.6091, 88.3633) (-130.9474, 88.409) (-131.2862, 88.453) (-131.6256, 88.4954) (-131.9656, 88.5362) (-132.3062, 88.5753) (-132.6472, 88.6128) (-132.9889, 88.6487) (-133.331, 88.683) (-133.6736, 88.7157) (-134.0168, 88.7468) (-134.3604, 88.7764) (-134.7046, 88.8044) (-135.0492, 88.8308) (-135.3943, 88.8557) (-135.7398, 88.879) (-136.0858, 88.9009) (-136.4322, 88.9212) (-136.7791, 88.94) (-137.1264, 88.9572) (-137.4741, 88.973) (-137.8222, 88.9873) (-138.1011, 88.9976) (-138.3104, 89.0046) (-138.45, 89.0089) (-138.5198, 89.011) knots 0 0 0 0 0 0 0.01428571 0.02857143 0.04285714 0.05714286 0.07142857 0.08571429 0.1 0.11428571 0.12857143 0.14285714 0.15714286 0.17142857 0.18571429 0.2 0.21428571 0.22857143 0.24285714 0.25714286 0.27142857 0.28571429 0.3 0.31428571 0.32857143 0.34285714 0.35714286 0.37142857 0.38571429 0.4 0.41428571 0.42857143 0.44285714 0.45714286 0.47142857 0.48571429 0.5 0.51428571 0.52857143 0.54285714 0.55714286 0.57142857 0.58571429 0.6 0.61428571 0.62857143 0.64285714 0.65714286 0.67142857 0.68571429 0.7 0.71428571 0.72857143 0.74285714 0.75714286 0.77142857 0.78571429 0.8 0.81428571 0.82857143 0.84285714 0.85714286 0.87142857 0.88571429 0.9 0.91428571 0.92857143 0.94285714 0.95714286 0.97142857 0.98571429 1 1 1 1 1 1
  arc A90 (-138.5198, 89.011) -> (-143.063, 81.142) centre (2.1352, 2.5578) ccw
  spline S45 degree 5 poles (-143.063, 81.142) (-143.0263, 81.0826) (-142.9527, 80.9639) (-142.8419, 80.7861) (-142.6937, 80.5498) (-142.5072, 80.2554) (-142.3197, 79.9622) (-142.1311, 79.6701) (-141.9414, 79.3791) (-141.7506, 79.0892) (-141.5587, 78.8005) (-141.3657, 78.5129) (-141.1716, 78.2265) (-140.9764, 77.9413) (-140.7801, 77.6572) (-140.5827, 77.3744) (-140.3841, 77.0928) (-140.1845, 76.8124) (-139.9837, 76.5332) (-139.7818, 76.2553) (-139.5788, 75.9787) (-139.3747, 75.7034) (-139.1694, 75.4293) (-138.963, 75.1565) (-138.7554, 74.8851) (-138.5467, 74.615) (-138.3368, 74.3463) (-138.1258, 74.0789) (-137.9136, 73.8129) (-137.7003, 73.5483) (-137.4857, 73.2851) (-137.27, 73.0234) (-137.0531, 72.7631) (-136.835, 72.5043) (-136.6157, 72.2471) (-136.3953, 71.9913) (-136.1736, 71.737) (-135.9506, 71.4844) (-135.7265, 71.2332) (-135.5011, 70.9837) (-135.2745, 70.7358) (-135.0466, 70.4896) (-134.8175, 70.2452) (-134.587, 70.0024) (-134.3552, 69.7615) (-134.1222, 69.5223) (-133.8878, 69.2849) (-133.6522, 69.0492) (-133.4153, 68.8154) (-133.177, 68.5834) (-132.9373, 68.3535) (-132.6962, 68.1257) (-132.4535, 67.9002) (-132.2093, 67.6769) (-131.9636, 67.4559) (-131.7165, 67.237) (-131.4681, 67.0201) (-131.2183, 66.8051) (-130.9672, 66.5923) (-130.7145, 66.3819) (-130.4599, 66.1745) (-130.2032, 65.9705) (-129.9443, 65.7703) (-129.683, 65.574) (-129.4198, 65.3809) (-129.155, 65.1903) (-128.8892, 65.0016) (-128.6223, 64.8146) (-128.354, 64.6303) (-128.083, 64.4509) (-127.8076, 64.2795) (-127.5823, 64.1513) (-127.41, 64.0613) (-127.2935, 64.0041) (-127.2349, 63.9763) knots -1 -1 -1 -1 -1 -1 -0.98571429 -0.97142857 -0.95714286 -0.94285714 -0.92857143 -0.91428571 -0.9 -0.88571429 -0.87142857 -0.85714286 -0.84285714 -0.82857143 -0.81428571 -0.8 -0.78571429 -0.77142857 -0.75714286 -0.74285714 -0.72857143 -0.71428571 -0.7 -0.68571429 -0.67142857 -0.65714286 -0.64285714 -0.62857143 -0.61428571 -0.6 -0.58571429 -0.57142857 -0.55714286 -0.54285714 -0.52857143 -0.51428571 -0.5 -0.48571429 -0.47142857 -0.45714286 -0.44285714 -0.42857143 -0.41428571 -0.4 -0.38571429 -0.37142857 -0.35714286 -0.34285714 -0.32857143 -0.31428571 -0.3 -0.28571429 -0.27142857 -0.25714286 -0.24285714 -0.22857143 -0.21428571 -0.2 -0.18571429 -0.17142857 -0.15714286 -0.14285714 -0.12857143 -0.11428571 -0.1 -0.08571429 -0.07142857 -0.05714286 -0.04285714 -0.02857143 -0.01428571 0 0 0 0 0 0
  line L45 (-127.2349, 63.9763) -> (-123.1504, 62.0365)
  arc A91 (-122.3896, 59.9381) -> (-123.1504, 62.0365) centre (-123.8314, 60.6025) ccw
  arc A92 (-122.3896, 59.9381) -> (-126.4911, 50.0361) centre (2.1352, 2.5578) ccw
  arc A93 (-128.5129, 49.0903) -> (-126.4911, 50.0361) centre (-127.9804, 50.5858) ccw
  line L46 (-128.5129, 49.0903) -> (-132.7727, 50.6069)
  spline S46 degree 5 poles (-132.7727, 50.6069) (-132.8339, 50.6286) (-132.9566, 50.6706) (-133.1421, 50.7288) (-133.392, 50.7974) (-133.708, 50.871) (-134.0265, 50.9358) (-134.3466, 50.9952) (-134.6674, 51.0517) (-134.9889, 51.1062) (-135.3108, 51.1586) (-135.6335, 51.2082) (-135.9571, 51.2541) (-136.2817, 51.2957) (-136.6075, 51.333) (-136.9341, 51.3663) (-137.2616, 51.3962) (-137.5897, 51.4233) (-137.9183, 51.4479) (-138.2473, 51.4702) (-138.5769, 51.4901) (-138.9069, 51.5076) (-139.2374, 51.5224) (-139.5685, 51.5345) (-139.9001, 51.5439) (-140.2321, 51.5508) (-140.5646, 51.5553) (-140.8975, 51.5575) (-141.2307, 51.5575) (-141.5643, 51.5553) (-141.8983, 51.5509) (-142.2325, 51.5444) (-142.5671, 51.5358) (-142.9021, 51.525) (-143.2373, 51.512) (-143.5728, 51.497) (-143.9086, 51.4799) (-144.2447, 51.4608) (-144.581, 51.4398) (-144.9175, 51.4168) (-145.2543, 51.3918) (-145.5913, 51.3649) (-145.9285, 51.3362) (-146.2659, 51.3055) (-146.6035, 51.273) (-146.9413, 51.2386) (-147.2792, 51.2023) (-147.6173, 51.1643) (-147.9556, 51.1244) (-148.294, 51.0828) (-148.6326, 51.0394) (-148.9713, 50.9942) (-149.3101, 50.9473) (-149.6491, 50.8987) (-149.9882, 50.8483) (-150.3273, 50.7963) (-150.6666, 50.7425) (-151.0059, 50.6871) (-151.3454, 50.63) (-151.6849, 50.5713) (-152.0245, 50.5109) (-152.3641, 50.4488) (-152.7038, 50.3852) (-153.0436, 50.3199) (-153.3834, 50.253) (-153.7233, 50.1846) (-154.0632, 50.1145) (-154.4031, 50.0429) (-154.743, 49.9697) (-155.0829, 49.8949) (-155.4229, 49.8186) (-155.6949, 49.7564) (-155.8989, 49.709) (-156.0349, 49.677) (-156.1029, 49.661) knots 0 0 0 0 0 0 0.01428571 0.02857143 0.04285714 0.05714286 0.07142857 0.08571429 0.1 0.11428571 0.12857143 0.14285714 0.15714286 0.17142857 0.18571429 0.2 0.21428571 0.22857143 0.24285714 0.25714286 0.27142857 0.28571429 0.3 0.31428571 0.32857143 0.34285714 0.35714286 0.37142857 0.38571429 0.4 0.41428571 0.42857143 0.44285714 0.45714286 0.47142857 0.48571429 0.5 0.51428571 0.52857143 0.54285714 0.55714286 0.57142857 0.58571429 0.6 0.61428571 0.62857143 0.64285714 0.65714286 0.67142857 0.68571429 0.7 0.71428571 0.72857143 0.74285714 0.75714286 0.77142857 0.78571429 0.8 0.81428571 0.82857143 0.84285714 0.85714286 0.87142857 0.88571429 0.9 0.91428571 0.92857143 0.94285714 0.95714286 0.97142857 0.98571429 1 1 1 1 1 1
  arc A94 (-156.1029, 49.661) -> (-158.4546, 40.8843) centre (2.1352, 2.5578) ccw
  spline S47 degree 5 poles (-158.4546, 40.8843) (-158.4037, 40.8364) (-158.3019, 40.7408) (-158.1489, 40.5977) (-157.9445, 40.4078) (-157.6883, 40.1717) (-157.4312, 39.937) (-157.1735, 39.7037) (-156.9149, 39.4717) (-156.6556, 39.2411) (-156.3955, 39.0118) (-156.1346, 38.784) (-155.873, 38.5576) (-155.6107, 38.3326) (-155.3475, 38.1091) (-155.0836, 37.887) (-154.819, 37.6663) (-154.5536, 37.4472) (-154.2874, 37.2295) (-154.0205, 37.0133) (-153.7528, 36.7987) (-153.4843, 36.5855) (-153.2151, 36.3739) (-152.9451, 36.1639) (-152.6743, 35.9554) (-152.4028, 35.7486) (-152.1306, 35.5433) (-151.8575, 35.3396) (-151.5837, 35.1376) (-151.3092, 34.9373) (-151.0338, 34.7386) (-150.7577, 34.5416) (-150.4809, 34.3463) (-150.2032, 34.1528) (-149.9248, 33.9611) (-149.6457, 33.7711) (-149.3657, 33.5829) (-149.085, 33.3965) (-148.8035, 33.2119) (-148.5212, 33.0292) (-148.2382, 32.8485) (-147.9543, 32.6696) (-147.6697, 32.4928) (-147.3843, 32.318) (-147.098, 32.1452) (-146.811, 31.9745) (-146.5232, 31.8058) (-146.2346, 31.6392) (-145.9452, 31.4746) (-145.655, 31.3123) (-145.364, 31.1522) (-145.0721, 30.9946) (-144.7794, 30.8396) (-144.4857, 30.6871) (-144.1912, 30.5372) (-143.8958, 30.3897) (-143.5997, 30.2445) (-143.3028, 30.1015) (-143.0052, 29.9609) (-142.7066, 29.8231) (-142.4071, 29.6886) (-142.1063, 29.558) (-141.8044, 29.4317) (-141.5012, 29.3097) (-141.1969, 29.1913) (-140.8919, 29.0757) (-140.5863, 28.9622) (-140.2801, 28.8507) (-139.9733, 28.7421) (-139.665, 28.6389) (-139.3546, 28.5447) (-139.1039, 28.4792) (-138.9141, 28.4368) (-138.7868, 28.4118) (-138.723, 28.4001) knots -1 -1 -1 -1 -1 -1 -0.98571429 -0.97142857 -0.95714286 -0.94285714 -0.92857143 -0.91428571 -0.9 -0.88571429 -0.87142857 -0.85714286 -0.84285714 -0.82857143 -0.81428571 -0.8 -0.78571429 -0.77142857 -0.75714286 -0.74285714 -0.72857143 -0.71428571 -0.7 -0.68571429 -0.67142857 -0.65714286 -0.64285714 -0.62857143 -0.61428571 -0.6 -0.58571429 -0.57142857 -0.55714286 -0.54285714 -0.52857143 -0.51428571 -0.5 -0.48571429 -0.47142857 -0.45714286 -0.44285714 -0.42857143 -0.41428571 -0.4 -0.38571429 -0.37142857 -0.35714286 -0.34285714 -0.32857143 -0.31428571 -0.3 -0.28571429 -0.27142857 -0.25714286 -0.24285714 -0.22857143 -0.21428571 -0.2 -0.18571429 -0.17142857 -0.15714286 -0.14285714 -0.12857143 -0.11428571 -0.1 -0.08571429 -0.07142857 -0.05714286 -0.04285714 -0.02857143 -0.01428571 0 0 0 0 0 0
  line L47 (-138.723, 28.4001) -> (-134.2756, 27.5835)
  arc A95 (-132.9976, 25.7536) -> (-134.2756, 27.5835) centre (-134.5623, 26.0221) ccw
  circle A96 centre (2.1352, 2.5578) radius 6.35
  circle A97 centre (2.1352, 2.5578) radius 6.35
  constraint concentric A0 A97
extrude "Extrude1'''" add sketch "Sketch2 (3)" along normal mid plane 100 separate body contours A96 A97 makes body 4 in component "Component'"
component "Spur Gear (24 teeth)" placed x (1, 0, 0) y (0, 1, 0) z (0, 0, 1) at (0, 0, 0)
component "Spur Gear (45 teeth)" placed x (0.884577, -0.466393, 0) y (0.466393, 0.884577, 0) z (0, 0, 1) at (-11.949, 436.1388, 0)
component "Component" placed x (1, 0, 0) y (0, 1, 0) z (0, 0, 1) at (0, 0, 0)
component "Component'" placed x (1, 0, 0) y (0, 1, 0) z (0, 0, 1) at (0, 0, 0)
